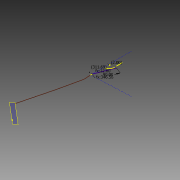
# Autodesk Inventor part: 1240x_Wire Depiction_V1
Saved by Autodesk Inventor 2020 (Build 240168000, 168)
## iProperties
Created: 2019-11-11
Part Number: 1240x_Wire Depiction_V1
Material: Copper
Document SubType Name: Modeling
Designer: RFLab
Density: 8.94 g/cm^3
Appearance: Copper - Satin
Author: RFLab
Autodesk Inventor part; units mm, degrees
ref_plane "YZ Plane" through (0, 0, 0) normal (1, 0, 0) x (0, 1, 0)
ref_plane "XZ Plane" through (0, 0, 0) normal (0, 1, 0) x (-1, 0, 0)
ref_plane "XY Plane" through (0, 0, 0) normal (0, 0, 1) x (1, 0, 0)
ref_plane "Work Plane1" through (0, 246.9812, -50.0427) normal (0, -0.1986, -0.9801) x (0.3752, -0.9085, 0.1841)
sketch "Sketch2" plane through (0, 246.9812, -50.0427) normal (0, -0.1986, -0.9801) x (0.3752, -0.9085, 0.1841)
  line L0 (1.8242, 3.8305) -> (-3.8305, 1.8242)
  line L1 (-3.8305, 1.8242) -> (-1.8242, -3.8305)
  line L2 (-1.8242, -3.8305) -> (3.8305, -1.8242)
  line L3 (3.8305, -1.8242) -> (1.8242, 3.8305)
  line L4 (-3.8305, 1.8242) -> (3.8305, -1.8242) construction
  point P0 (233.5906, 94.5486)
  point P1 (0, 0)
  point P2 (0, 0)
  dimension "d7" = 6
  dimension "d9" = 6
  constraints: 10 end point, 2 parallel, 1 coincident, 1 midpoint, 1 perpendicular
  measures "d7" distance of L0.start L0.end
  measures "d9" distance of L0.end L1.end
sketch "Sketch1" plane through (0, 0, 0) normal (1, 0, 0) x (0, 1, 0)
  circle A0 centre (0, 0) radius 249 construction
  circle A1 centre (0, 0) radius 252 construction
  circle A2 centre (107.5, -817.5) radius 12.7 construction
  circle A3 centre (107.5, -817.5) radius 14.5 construction
  circle A4 centre (74.5, -817.5) radius 14.5 construction
  circle A5 centre (74.5, -817.5) radius 12.7 construction
  circle A6 centre (40, -1342.5) radius 40 construction
  line L0 (7.5, -1515.8) -> (7.5, -1459.2) construction
  line L1 (0.5, -1515.8) -> (0.5, -1459.2) construction
  circle A7 centre (40, -1342.5) radius 43 construction
  line L2 (7.5, -1459.2) -> (0.5, -1459.2) construction
  line L3 (7.5, -1487.5) -> (0.5, -1487.5) construction
  line L4 (4, -1459.2) -> (4, -1487.5)
  line L5 (4, -1459.2) -> (-2.3093, -1334.824)
  circle A8 centre (107.5, -817.5) radius 15.7 construction
  line L6 (246.9812, -50.0427) -> (92.1127, -814.3823)
  line L7 (92.1127, -814.3823) -> (-2.3093, -1334.824)
sweep "Sweep1" add profiles "Sketch2" path "Sketch1"
ref_plane "Work Plane2" through (0.425, 4.5, -1487.5) normal (0, -1, 0) x (1, 0, 0)
sketch "Sketch3" plane through (2.8662, 4.5, -1459.1207) normal (0, 1, 0) x (1, 0, 0)
  line L0 (-5.9943, 0.0066) -> (0, 0) projected
  line L1 (0, 0) -> (0, 28.3793) projected
  line L2 (-5.9943, 28.3793) -> (0, 28.3793) projected
  line L3 (-5.9943, 0.0066) -> (-5.9943, 28.3793) projected
  line L4 (-405.574, 755.2769) -> (-292.3211, 735.3073) projected
  line L5 (0.2618, 0.1519) -> (-5.7324, 0.1586) projected
  line L6 (-2.7353, 0.1553) -> (-2.7353, 774.7681) construction
  line L7 (-2.7353, 0.1553) -> (771.8776, 0.1553) construction
  line L8 (0, 28.3793) -> (-5.9943, 28.3793) projected
  line L9 (-2.7353, 28.3793) -> (212.7395, 476.7703)
  arc A0 (-512.9326, 851.3967) -> (-442.0119, 761.7018) centre (-427.0782, 846.3953) ccw projected
  point P0 (-2.8662, -1459.1207)
  dimension "d12" = 90
  dimension "d13" = 260
  dimension "d14" = 25.667
  dimension "LengthExtension" = 497.4775
  constraints: 6 end point, 1 horizontal, 1 midpoint, 1 perpendicular, 1 point on line, 2 other
  measures "d12" angle of L7 L6
  measures "d14" angle of L6 L9
  measures "LengthExtension" distance of L9.start L9.end
sketch "Sketch4" plane through (2.8662, 7.1281, -1487.5) normal (0, 0, -1) x (-0.999, -0.0436, 0)
  line L0 (-0.8742, 0.3341) -> (-50.8266, -1.8479) projected
  line L1 (6, 0) -> (0, 0) projected
  line L2 (0, 0) -> (0, -6) projected
  line L3 (0, -6) -> (6, -6) projected
  line L4 (6, -6) -> (6, 0) projected
  point P0 (3.1746, -6.9962)
sweep "Sweep2" add profiles "Sketch4" path "Sketch3" separate body path curves L9
equation "\"LengthExtension\" = d16"
equation "\"d16\" = 497.477531"
body "Solid1"
body "Solid2"
